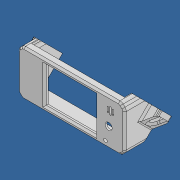
# Autodesk Inventor part: Print_Parts_TFT
Saved by Autodesk Inventor 2020 (Build 240168000, 168)
## iProperties
Created: 2020-11-15
Part Number: Print_Parts_TFT
Material: 一般
Document SubType Name: Modeling
Designer: kenta iguchi
Density: 1 g/cm^3
Appearance: 既定
Author: kenta iguchi
Autodesk Inventor part; units mm, degrees
ref_plane "YZ Plane" through (0, 0, 0) normal (1, 0, 0) x (0, 1, 0)
ref_plane "XZ Plane" through (0, 0, 0) normal (0, 1, 0) x (-1, 0, 0)
ref_plane "XY Plane" through (0, 0, 0) normal (0, 0, 1) x (1, 0, 0)
sketch "スケッチ1" plane through (0, 0, 0) normal (0, 0, 1) x (1, 0, 0)
  line L0 (28.75, -20.25) -> (-28.75, -20.25)
  line L1 (-28.75, -20.25) -> (-28.75, 20.25)
  line L2 (-28.75, 20.25) -> (28.75, 20.25)
  line L3 (28.75, 20.25) -> (28.75, -20.25)
  line L4 (28.75, -20.25) -> (-28.75, 20.25) construction
  line L5 (-28.75, -20.25) -> (28.75, 20.25) construction
  line L6 (-51.1, -23) -> (53.9, -23)
  line L7 (53.9, -23) -> (53.9, 23)
  line L8 (53.9, 23) -> (-51.1, 23)
  line L9 (-51.1, 23) -> (-51.1, -23)
  line L10 (-51.1, -23) -> (53.9, 23) construction
  line L11 (53.9, -23) -> (-51.1, 23) construction
  point P0 (0, 0)
  point P1 (1.4, 0)
  point P2 (1.4, 0)
  point P3 (0, 0)
  dimension "d0" = 40.5
  dimension "d1" = 57.5
  dimension "d2" = 51.1
  dimension "d4" = 53.9
  dimension "d5" = 46
  constraints: 24 end point, 6 midpoint, 4 parallel, 2 horizontal, 2 perpendicular, 1 horizontal alignment
  measures "d0" distance of L2.end L0.start
  measures "d1" distance of L0.start L0.end
  measures "d2" distance from line of point (0, 0) L9
  measures "d4" distance from line of L7 point (0, 0)
  measures "d5" distance of L6.end L7.end
extrude "押し出し1" add sketch "スケッチ1" against normal blind 4
sketch "スケッチ2" plane through (0, 0, 0) normal (0, 0, 1) x (1, 0, 0)
  line L0 (53.9, 23) -> (-51.1, 23) projected
  line L1 (-48.64, 20.575) -> (51.44, 20.575)
  line L2 (51.44, 20.575) -> (51.44, -20.575)
  line L3 (51.44, -20.575) -> (-48.64, -20.575)
  line L4 (-48.64, -20.575) -> (-48.64, 20.575)
  line L5 (-51.1, 23) -> (53.9, 23) projected
  point P0 (0, 0)
  point P1 (51.44, 0)
  point P2 (1.4, 23)
  point P3 (1.4, 20.575)
  point P4 (1.4, 23)
  dimension "d8" = 100.08
  dimension "d9" = 41.15
  constraints: 8 end point, 4 midpoint, 2 parallel, 1 horizontal, 1 horizontal alignment, 1 perpendicular, 1 vertical alignment
  measures "d8" distance of L2.end L3.end
  measures "d9" distance of L1.end L2.end
hole "穴1" at (51.44, 20.575, 0) at (51.44, -20.575, 0) at (-48.64, -20.575, 0) at (-48.64, 20.575, 0) direction (0, 0, -1) diameter 4.3 depth 8 tip angle 118
sketch "スケッチ3" plane through (0, 0, 0) normal (0, 0, 1) x (1, 0, 0)
  line L0 (53.9, -23) -> (53.9, 23) projected
  circle A0 centre (40.44, -19.31) radius 2
  line L1 (-51.1, -23) -> (53.9, -23) projected
  point P0 (0, 0)
  dimension "d18" = 13.46
  dimension "d19" = 4
  dimension "d26" = 3.69
  constraints: 1 centre point, 1 coincident
  measures "d18" distance from line of point (40.44, -19.31) L0
  measures "d19" diameter of A0
  measures "d26" distance from line of point (40.44, -19.31) L1
extrude "押し出し2" cut sketch "スケッチ3" against normal blind 10
sketch "スケッチ4" plane through (0, 0, -4) normal (0, 0, -1) x (-1, 0, 0)
  circle A0 centre (-40.44, -19.31) radius 2 projected
  line L0 (-37.34, -16.21) -> (-43.54, -16.21)
  line L1 (-43.54, -16.21) -> (-43.54, -22.41)
  line L2 (-43.54, -22.41) -> (-37.34, -22.41)
  line L3 (-37.34, -22.41) -> (-37.34, -16.21)
  line L4 (-37.34, -16.21) -> (-43.54, -22.41) construction
  line L5 (-43.54, -16.21) -> (-37.34, -22.41) construction
  point P0 (0, 0)
  dimension "d22" = 6.2
  dimension "d23" = 6.2
  constraints: 12 end point, 2 midpoint, 2 parallel, 1 horizontal, 1 perpendicular
  measures "d22" distance of L2.end L1.end
  measures "d23" distance of L1.end L0.end
extrude "押し出し3" cut sketch "スケッチ4" against normal blind 1
sketch "スケッチ5" plane through (0, 0, 0) normal (0, 0, 1) x (1, 0, 0)
  line L0 (-51.1, -23) -> (53.9, -23) projected
  line L1 (53.9, -23) -> (53.9, 23) projected
  circle A0 centre (44.08, -3.68) radius 4
  point P0 (0, 0)
  dimension "d27" = 19.32
  dimension "d28" = 9.82
  dimension "d29" = 8
  constraints: 1 centre point, 1 coincident
  measures "d27" distance from line of point (44.08, -3.68) L0
  measures "d28" distance from line of point (44.08, -3.68) L1
  measures "d29" diameter of A0
extrude "押し出し4" cut sketch "スケッチ5" against normal through all
chamfer "面取り1" distance 2 angle 45 4 edges at (-28.75, 0, 0) (0, 20.25, 0) (28.75, 0, 0) (0, -20.25, 0)
sketch "スケッチ6" plane through (0, 0, -4) normal (0, 0, -1) x (-1, 0, 0)
  circle A0 centre (-44.08, -3.68) radius 4 projected
  line L0 (-50.58, -10.18) -> (-37.58, -10.18)
  line L1 (-37.58, -10.18) -> (-37.58, 2.82)
  line L2 (-37.58, 2.82) -> (-50.58, 2.82)
  line L3 (-50.58, 2.82) -> (-50.58, -10.18)
  line L4 (-50.58, -10.18) -> (-37.58, 2.82) construction
  line L5 (-37.58, -10.18) -> (-50.58, 2.82) construction
  point P0 (0, 0)
  dimension "d35" = 13
  dimension "d36" = 13
  constraints: 12 end point, 2 midpoint, 2 parallel, 1 horizontal, 1 perpendicular
  measures "d35" distance of L2.end L1.end
  measures "d36" distance of L1.end L0.end
extrude "押し出し5" cut sketch "スケッチ6" against normal blind 2
sketch "スケッチ7" plane through (0, 0, 0) normal (0, 0, 1) x (1, 0, 0)
  line L0 (53.9, 23) -> (-51.1, 23)
  line L1 (53.9, -23) -> (53.9, 23)
  circle A0 centre (46.09, 12.41) radius 4.5
  line L2 (46.09, 16.91) -> (46.09, 7.91) construction
  line L3 (45.34, 16.16) -> (45.34, 8.66)
  line L4 (46.84, 8.66) -> (46.84, 16.16)
  arc A1 (46.84, 16.16) -> (45.34, 16.16) centre (46.09, 16.16) ccw
  arc A2 (45.34, 8.66) -> (46.84, 8.66) centre (46.09, 8.66) ccw
  line L5 (43.09, 15.764102) -> (43.09, 9.055898) construction
  line L6 (42.34, 15.014102) -> (42.34, 9.805898)
  line L7 (43.84, 9.805898) -> (43.84, 15.014102)
  arc A3 (43.84, 15.014102) -> (42.34, 15.014102) centre (43.09, 15.014102) ccw
  arc A4 (42.34, 9.805898) -> (43.84, 9.805898) centre (43.09, 9.805898) ccw
  line L8 (49.09, 15.764102) -> (49.09, 9.055898) construction
  line L9 (48.34, 15.014102) -> (48.34, 9.805898)
  line L10 (49.84, 9.805898) -> (49.84, 15.014102)
  arc A5 (49.84, 15.014102) -> (48.34, 15.014102) centre (49.09, 15.014102) ccw
  arc A6 (48.34, 9.805898) -> (49.84, 9.805898) centre (49.09, 9.805898) ccw
  point P0 (0, 0)
  point P1 (43.09, 12.41)
  point P2 (49.09, 12.41)
  dimension "d39" = 7.81
  dimension "d40" = 10.59
  dimension "d41" = 9
  dimension "d42" = 1.5
  dimension "d43" = 1.5
  dimension "d44" = 1.5
  dimension "d45" = 3
  dimension "d46" = 6
  constraints: 24 end point, 24 point on circle, 12 tangent, 7 centre point, 6 point on line, 4 parallel, 3 midpoint, 2 coincident, 2 vertical
  measures "d39" distance from line of point (46.09, 12.41) L1
  measures "d40" distance from line of point (46.09, 12.41) L0
  measures "d41" diameter of A0
  measures "d42" diameter of A2
  measures "d43" diameter of A4
  measures "d44" diameter of A6
  measures "d45" distance of A0.centre point (43.09, 12.41)
  measures "d46" distance between parallel lines of L8 L5
extrude "押し出し6" cut sketch "スケッチ7" against normal blind 10 contours L10 A0 A6 L9 A5 | A0 A5 L10 | L10 A6 A0 | A1 L4 A2 L3 | A3 L7 A4 A0 L6 | A0 L6 A3 | A4 L6 A0
sketch "スケッチ8" plane through (0, 0, -4) normal (0, 0, -1) x (-1, 0, 0)
  line L0 (-48.34, 15.014102) -> (-48.34, 9.805898)
  arc A0 (-49.84, 9.805898) -> (-48.34, 9.805898) centre (-49.09, 9.805898) ccw
  line L1 (-49.84, 9.805898) -> (-49.84, 15.014102)
  arc A1 (-48.34, 15.014102) -> (-49.84, 15.014102) centre (-49.09, 15.014102) ccw
  line L2 (-46.84, 8.66) -> (-46.84, 16.16)
  arc A2 (-45.34, 16.16) -> (-46.84, 16.16) centre (-46.09, 16.16) ccw
  line L3 (-45.34, 16.16) -> (-45.34, 8.66)
  arc A3 (-46.84, 8.66) -> (-45.34, 8.66) centre (-46.09, 8.66) ccw
  line L4 (-42.34, 15.014102) -> (-42.34, 9.805898)
  arc A4 (-43.84, 9.805898) -> (-42.34, 9.805898) centre (-43.09, 9.805898) ccw
  line L5 (-43.84, 9.805898) -> (-43.84, 15.014102)
  arc A5 (-42.34, 15.014102) -> (-43.84, 15.014102) centre (-43.09, 15.014102) ccw
  line L6 (-46.09, 8.66) -> (-46.09, 16.16)
  circle A6 centre (-46.09, 12.41) radius 5
  point P0 (0, 0)
  dimension "d49" = 10
  constraints: 2 end point, 1 centre point, 1 coincident, 1 midpoint, 1 vertical
  measures "d49" diameter of A6
extrude "押し出し7" cut sketch "スケッチ8" against normal blind 2
sketch "スケッチ9" plane through (0, 0, 0) normal (0, 0, 1) x (1, 0, 0)
  line L0 (53.9, 23) -> (-51.1, 23) projected
  line L1 (-51.1, 23) -> (-51.1, -23) projected
  line L2 (-51.1, -23) -> (53.9, -23) projected
  line L3 (53.9, -23) -> (53.9, 23) projected
  line L4 (-54.1, 26) -> (56.9, 26)
  line L5 (56.9, 26) -> (56.9, -26)
  line L6 (56.9, -26) -> (-54.1, -26)
  line L7 (-54.1, -26) -> (-54.1, 26)
  circle A0 centre (51.44, 20.575) radius 2.15 projected
  circle A1 centre (51.44, 20.575) radius 4
  point P0 (0, 0)
  dimension "d52" = 3
  dimension "d67" = 8
  constraints: 8 end point, 1 centre point, 1 coincident, 3 other
  measures "d52" distance between parallel lines of L0 L4
  measures "d67" diameter of A1
extrude "押し出し8" add sketch "スケッチ9" against normal up to surface (4 mm away) contours L0 A1 L3 | L4 L5 L6 L7 picked at (50.3712, 23.236403)
sketch "スケッチ10" plane through (0, 0, -4) normal (0, 0, -1) x (-1, 0, 0)
  circle A0 centre (48.64, -20.575) radius 2.15 projected
  circle A1 centre (-51.44, 20.575) radius 2.15 projected
  circle A2 centre (48.64, 20.575) radius 2.15 projected
  circle A3 centre (-51.44, 20.575) radius 2.2
  circle A4 centre (48.64, 20.575) radius 2.2
  circle A5 centre (48.64, -20.575) radius 2.2
  circle A6 centre (-51.44, -20.575) radius 2.15 projected
  circle A7 centre (-51.44, -20.575) radius 2.2
  circle A8 centre (-51.44, 20.575) radius 2.15 projected
  circle A9 centre (-51.44, 20.575) radius 4
  circle A10 centre (48.64, 20.575) radius 4
  circle A11 centre (48.64, -20.575) radius 4
  circle A12 centre (-51.44, -20.575) radius 4
  point P0 (0, 0)
  dimension "d55" = 4.4
  dimension "d56" = 4.4
  dimension "d57" = 4.4
  dimension "d58" = 4.4
  dimension "d59" = 8
  dimension "d60" = 8
  dimension "d61" = 8
  dimension "d62" = 8
  constraints: 8 centre point, 8 coincident
  measures "d55" diameter of A3
  measures "d56" diameter of A4
  measures "d57" diameter of A5
  measures "d58" diameter of A7
  measures "d59" diameter of A9
  measures "d60" diameter of A10
  measures "d61" diameter of A11
  measures "d62" diameter of A12
extrude "押し出し9" add sketch "スケッチ10" along normal blind 3 contours A9 | A10 | A11 | A12
sketch "スケッチ11" plane through (0, 0, 0) normal (0, 0, 1) x (1, 0, 0)
  circle A0 centre (-48.64, 20.575) radius 2.15 projected
  circle A1 centre (51.44, -20.575) radius 2.15 projected
  circle A2 centre (51.44, 20.575) radius 2.15 projected
  circle A3 centre (-48.64, -20.575) radius 2.15 projected
  point P0 (0, 0)
extrude "押し出し10" add sketch "スケッチ11" against normal up to surface (4 mm away)
sketch "スケッチ12" plane through (0, 0, -4) normal (0, 0, -1) x (-1, 0, 0)
  circle A0 centre (48.64, 20.575) radius 4 projected
  circle A1 centre (-51.44, 20.575) radius 4 projected
  circle A2 centre (48.64, -20.575) radius 4 projected
  circle A3 centre (-51.44, -20.575) radius 4 projected
  line L0 (54.1, 26) -> (54.1, -26) projected
  line L1 (-56.9, 26) -> (54.1, 26) projected
  line L2 (-56.9, -26) -> (-56.9, 26) projected
  line L3 (54.1, -26) -> (-56.9, -26) projected
  line L4 (51.3, 23.2) -> (51.3, -23.2)
  line L5 (51.3, -23.2) -> (-54.1, -23.2)
  line L6 (-54.1, -23.2) -> (-54.1, 23.2)
  line L7 (-54.1, 23.2) -> (51.3, 23.2)
  circle A4 centre (-51.44, 20.575) radius 4 projected
  circle A5 centre (-51.44, 20.575) radius 2.2 projected
  circle A6 centre (48.64, 20.575) radius 2.2 projected
  circle A7 centre (48.64, -20.575) radius 2.2 projected
  circle A8 centre (-51.44, -20.575) radius 2.2 projected
  point P0 (0, 0)
  point P1 (-48.421826, 23.2)
  point P2 (45.621826, 23.2)
  point P3 (51.3, 17.587627)
  point P4 (51.3, -17.587627)
  point P5 (45.621826, -23.2)
  point P6 (-48.421826, -23.2)
  point P7 (-54.1, -17.587627)
  point P8 (-54.1, 17.587627)
  dimension "d68" = 2.8
  constraints: 8 end point, 3 other
  measures "d68" distance between parallel lines of L1 L7
extrude "押し出し11" add sketch "スケッチ12" along normal blind 4 contours L0 L3 L2 L1
sketch "スケッチ13" plane through (51.44, 20.575, -4) normal (0, 0, -1) x (-1, 0, 0)
  circle A0 centre (0, 0) radius 2.2 projected
  circle A1 centre (0, -41.15) radius 2.2 projected
  circle A2 centre (100.08, -41.15) radius 2.2 projected
  circle A3 centre (100.08, 0) radius 2.2 projected
  point P0 (51.44, -20.575)
extrude "押し出し12" cut sketch "スケッチ13" against normal blind 2
sketch "スケッチ14" plane through (0, 0, -8) normal (0, 0, -1) x (-1, 0, 0)
  line L0 (54.1, -26) -> (54.1, 26)
  line L1 (-56.9, 26) -> (-56.9, -26)
  line L2 (-54.1, -17.587627) -> (-54.1, 17.587627)
  line L3 (51.3, 17.587627) -> (51.3, -17.587627)
  line L4 (-56.9, 26) -> (54.1, 26)
  line L5 (54.1, 26) -> (59.3, 26)
  line L6 (59.3, 26) -> (59.3, -26)
  line L7 (59.3, -26) -> (54.1, -26)
  line L8 (54.1, -26) -> (54.1, 26)
  line L9 (-56.9, 26) -> (-62.1, 26)
  line L10 (-62.1, 26) -> (-62.1, -26)
  line L11 (-62.1, -26) -> (-56.9, -26)
  line L12 (-56.9, -26) -> (-56.9, 26)
  point P0 (0, 0)
  point P1 (-56.9, -26)
  dimension "d80" = 8
  dimension "d81" = 8
  constraints: 16 end point, 4 parallel, 2 horizontal, 2 perpendicular, 1 coincident, 1 horizontal alignment, 1 point on line
  measures "d80" distance between parallel lines of L6 L3
  measures "d81" distance between parallel lines of L10 L2
extrude "押し出し13" add sketch "スケッチ14" against normal up to surface (8 mm away)
sketch "スケッチ16" plane through (0, 0, -8) normal (0, 0, -1) x (-1, 0, 0)
  line L0 (59.3, 26) -> (-62.1, 26)
  line L1 (-62.1, 26) -> (-62.1, -26)
  line L2 (-62.1, -26) -> (59.3, -26)
  line L3 (59.3, -26) -> (59.3, 26)
  arc A0 (45.621826, -23.2) -> (51.3, -17.587627) centre (48.64, -20.575) ccw
  arc A1 (-54.1, -17.587627) -> (-48.421826, -23.2) centre (-51.44, -20.575) ccw
  line L4 (-54.1, -17.587627) -> (-54.1, 17.587627)
  arc A2 (-48.421826, 23.2) -> (-54.1, 17.587627) centre (-51.44, 20.575) ccw
  arc A3 (51.3, 17.587627) -> (45.621826, 23.2) centre (48.64, 20.575) ccw
  line L5 (51.3, 17.587627) -> (51.3, -17.587627)
  line L6 (-62.1, 26) -> (-54.1, 26)
  line L7 (-54.1, 26) -> (-54.1, -26)
  line L8 (-54.1, -26) -> (-62.1, -26)
  line L9 (-62.1, -26) -> (-62.1, 26)
  line L10 (-62.1, 26) -> (59.3, 26)
  line L11 (59.3, 26) -> (51.3, 26)
  line L12 (51.3, 26) -> (51.3, -26)
  line L13 (51.3, -26) -> (59.3, -26)
  line L14 (59.3, -26) -> (59.3, 26)
  point P0 (0, 0)
  point P1 (51.3, -23.562373)
  point P2 (51.3, 23.562373)
  point P3 (-54.1, 23.562373)
  point P4 (-54.1, -23.562373)
  constraints: 16 end point, 4 parallel, 2 horizontal, 2 perpendicular, 2 point on line, 2 vertical alignment
extrude "押し出し14" add sketch "スケッチ16" along normal blind 10 contours L3 L2 L12 A0 L5 A3 L0 | L7 A2 L4 A1 L2 L1 L0
chamfer "面取り4" distance 2 angle 45 2 edges at (58.1, 26, -18) (-55.3, 26, -18)
sketch "スケッチ17" plane through (-59.3, -26, 0) normal (-1, 0, 0) x (0, 0, 1)
  line L0 (-18, 50) -> (-16, 52) projected
  line L1 (-18, 0) -> (-18, 50) projected
  line L2 (0, 0) -> (-18, 0) projected
  line L3 (-18, 50) -> (-68, 0)
  line L4 (-8, 0) -> (-18, 0) projected
  line L5 (-68, 0) -> (-18, 0)
  line L6 (-18, 0) -> (0, 0) projected
  line L7 (-18, 0) -> (-43, 25)
  point P0 (0, 26)
  constraints: 6 end point, 2 collinear, 1 midpoint
extrude "押し出し15" add sketch "スケッチ17" against normal up to surface (8 mm away) contours L7 L3 L1
sketch "スケッチ18" plane through (62.1, -26, 0) normal (1, 0, 0) x (0, 0, -1)
  line L0 (18, 50) -> (18, 0)
  line L1 (4, 8.412373) -> (4, 43.587627)
  line L2 (7, 8.412373) -> (4, 8.412373)
  line L3 (7, 8.412373) -> (18, 8.412373)
  line L4 (18, 2.437627) -> (18, 8.412373)
  line L5 (8, 2.437627) -> (18, 2.437627)
  line L6 (8, 0) -> (18, 0)
  line L7 (43, 25) -> (18, 0)
  line L8 (16, 52) -> (43, 25)
  line L9 (18, 43.587627) -> (18, 49.562373)
  line L10 (7, 43.587627) -> (18, 43.587627)
  line L11 (4, 43.587627) -> (7, 43.587627)
  line L12 (8, 0) -> (8, 2.437627)
  line L13 (8, 52) -> (16, 52)
  line L14 (8, 49.562373) -> (8, 52)
  line L15 (8, 49.562373) -> (18, 49.562373)
  point P0 (0, 26)
  point P1 (18, 50)
  point P2 (18, 8.412373)
  point P3 (18, 0)
extrude "押し出し16" add sketch "スケッチ18" against normal up to surface (8 mm away) contours L8 L7 L0
sketch "スケッチ20" plane through (-59.3, -26, 0) normal (-1, 0, 0) x (0, 0, 1)
  line L0 (0, 0) -> (-18, 0) projected
  line L1 (0, 0) -> (0, 52) projected
  line L2 (-8.6, 38.36) -> (-11.5, 38.36)
  line L3 (-11.5, 38.36) -> (-11.5, 11.86)
  line L4 (-11.5, 11.86) -> (-8.6, 11.86)
  line L5 (-8.6, 11.86) -> (-8.6, 38.36)
  point P0 (0, 26)
  dimension "d96" = 8.6
  dimension "d97" = 2.9
  dimension "d98" = 11.86
  dimension "d99" = 38.36
  constraints: 8 end point, 2 parallel, 1 horizontal, 1 perpendicular
  measures "d96" distance between parallel lines of L1 L5
  measures "d97" distance of L3.end L4.end
  measures "d98" distance between parallel lines of L0 L4
  measures "d99" distance between parallel lines of L0 L2
extrude "押し出し18" cut sketch "スケッチ20" against normal blind 10
sketch "スケッチ21" plane through (-59.3, -26, 0) normal (-1, 0, 0) x (0, 0, 1)
  line L0 (-8.6, 38.36) -> (-8.6, 11.86) projected
  line L1 (-8.6, 11.86) -> (-11.5, 11.86) projected
  line L2 (-11.5, 11.86) -> (-11.5, 38.36) projected
  line L3 (-11.5, 38.36) -> (-8.6, 38.36) projected
  line L4 (-12.5, 10.86) -> (-7.6, 10.86)
  line L5 (-7.6, 10.86) -> (-7.6, 39.36)
  line L6 (-7.6, 39.36) -> (-12.5, 39.36)
  line L7 (-12.5, 39.36) -> (-12.5, 10.86)
  point P0 (0, 26)
  dimension "d102" = 1
  constraints: 8 end point, 3 other
  measures "d102" distance between parallel lines of L1 L4
extrude "押し出し19" cut sketch "スケッチ21" against normal blind 10
fillet "フィレット2" radius 1 4 edges at (-55.3, 13.36, -12.5) (-55.3, 13.36, -7.6) (-55.3, -15.14, -12.5) (-55.3, -15.14, -7.6)
sketch "スケッチ24" plane through (62.1, 26, -16) normal (0, 0.7071068, -0.7071068) x (-1, 0, 0)
  line L0 (0, 0) -> (0, -38.183766)
  line L1 (0, -38.183766) -> (-12, -38.183766)
  line L2 (-12, -38.183766) -> (-12, -18.183766)
  line L3 (-12, -18.183766) -> (0, -18.183766)
  line L4 (0, -18.183766) -> (0, -38.183766)
  line L5 (113.4, 0) -> (113.4, -38.183766)
  line L6 (121.4, -38.183766) -> (121.4, 0)
  line L7 (121.4, 0) -> (113.4, 0)
  line L8 (121.4, -38.183766) -> (121.4, 0)
  line L9 (121.4, -38.183766) -> (133.4, -38.183766)
  line L10 (133.4, -38.183766) -> (133.4, -18.183766)
  line L11 (133.4, -18.183766) -> (121.4, -18.183766)
  line L12 (121.4, -18.183766) -> (121.4, -38.183766)
  line L13 (121.4, -38.183766) -> (113.4, -38.183766)
  point P0 (62.1, -7.071068)
  point P1 (0, -18.183766)
  point P2 (8, -38.183766)
  dimension "d118" = 12
  dimension "d119" = 20
  dimension "d120" = 12
  dimension "d121" = 20
  constraints: 16 end point, 4 parallel, 2 horizontal, 2 horizontal alignment, 2 perpendicular
  measures "d118" distance of L2.end L3.end
  measures "d119" distance of L1.end L2.end
  measures "d120" distance of L11.end L10.end
  measures "d121" distance of L10.end L9.end
extrude "押し出し21" add sketch "スケッチ24" against normal blind 5 contours L0 L1 L2 L3 | L6 L11 L10 L9
chamfer "面取り6" distance 12 angle 45 2 edges at (62.1, 2.5355, -32.3934) (-59.3, 2.5355, -32.3934)
chamfer "面取り7" distance 5 angle 45 4 edges at (62.1, -26, -9) (-59.3, -26, -9) (62.1, 26, -8) (-59.3, 26, -8)
fillet "フィレット3" radius 5 8 edges at (-59.3, 21, -10.5) (-54.3, 26, -8) (-59.3, -21, -11.5) (-54.3, -26, -9) (57.1, -26, -9) (62.1, -21, -11.5) (62.1, 21, -10.5) (57.1, 26, -8)
chamfer "面取り8" distance 2 angle 45 8 edges at (74.1, 9.6066, -25.3223) (74.1, 11.3744, -27.0901) (74.1, -4.5355, -39.4645) (74.1, -2.7678, -41.2322) (-71.3, 9.6066, -25.3223) (-71.3, 11.3744, -27.0901) (-71.3, -4.5355, -39.4645) (-71.3, -2.7678, -41.2322)
fillet "フィレット4" radius 2 12 edges at (-59.3, -5.9497, -23.9082) (62.1, -5.9497, -23.9082) (72.1, 10.6673, -26.383) (74.1, 9.9602, -28.5043) (74.1, -1.3536, -39.818) (72.1, -3.4748, -40.5252) (-69.3, -3.4748, -40.5252) (-71.3, -1.3536, -39.818) (-71.3, 9.9602, -28.5043) (-69.3, 10.6673, -26.383) (62.1, 7.1318, -22.8475) (-59.3, 7.1318, -22.8475)
chamfer "面取り9" distance 2 angle 45 16 edges at (-58.9194, 20.8423, 0) (-56.8, 23.5, 0) (-54.1423, 25.6194, 0) (1.4, 26, 0) (56.9423, 25.6194, 0) (59.6, 23.5, 0) (61.7194, 20.8423, 0) (62.1, 0, 0) (61.7194, -20.8423, 0) (59.6, -23.5, 0) (56.9423, -25.6194, 0) (1.4, -26, 0) (-54.1423, -25.6194, 0) (-56.8, -23.5, 0) (-58.9194, -20.8423, 0) (-59.3, 0, 0)
sketch "スケッチ26" plane through (51.44, 20.575, -18) normal (0, 0, 1) x (1, 0, 0)
  arc A0 (2.66, -2.987373) -> (2.66, 2.987373) centre (0, 0) ccw
  line L0 (2.66, 2.987373) -> (2.66, -2.987373)
  arc A1 (2.66, -44.137373) -> (2.66, -38.162627) centre (0, -41.15) ccw
  line L1 (2.66, -38.162627) -> (2.66, -44.137373)
  arc A2 (-102.74, 2.987373) -> (-102.74, -2.987373) centre (-100.08, 0) ccw
  line L2 (-102.74, -2.987373) -> (-102.74, 2.987373)
  arc A3 (-102.74, -38.162627) -> (-102.74, -44.137373) centre (-100.08, -41.15) ccw
  line L3 (-102.74, -44.137373) -> (-102.74, -38.162627)
  point P0 (-51.44, -20.575)
extrude "押し出し22" cut sketch "スケッチ26" against normal blind 10
sketch "スケッチ27" plane through (0, 0, -8) normal (0, 0, -1) x (-1, 0, 0)
  line L0 (51.3, -26) -> (51.3, -23.562373)
  arc A0 (45.621826, -23.2) -> (51.3, -23.562373) centre (48.64, -20.575) ccw
  line L1 (45.621826, -23.2) -> (-48.421826, -23.2)
  arc A1 (-54.1, -23.562373) -> (-48.421826, -23.2) centre (-51.44, -20.575) ccw
  line L2 (-54.1, -23.562373) -> (-54.1, -26)
  line L3 (-54.1, -26) -> (51.3, -26)
  point P0 (0, 0)
extrude "押し出し23" add sketch "スケッチ27" along normal up to surface surface through (62.1, -1, -43) normal (0, -0.7071068, -0.7071068)
ref_plane "作業平面2" through (-61.3, -1, -14.715729) normal (0, 0.7071068, -0.7071068) x (-1, 0, 0)
sketch "スケッチ29" plane through (-61.3, -1, -14.715729) normal (0, 0.7071068, -0.7071068) x (-1, 0, 0)
  arc A0 (8.585786, -0.585786) -> (7.171573, 0) centre (7.171573, -2) ccw
  line L0 (9.414214, -1.414214) -> (8.585786, -0.585786)
  arc A1 (10, -2.828427) -> (9.414214, -1.414214) centre (8, -2.828427) ccw
  line L1 (10, -2.828427) -> (10, -17.171573)
  arc A2 (9.414214, -18.585786) -> (10, -17.171573) centre (8, -17.171573) ccw
  line L2 (8.585786, -19.414214) -> (9.414214, -18.585786)
  arc A3 (7.171573, -20) -> (8.585786, -19.414214) centre (7.171573, -18) ccw
  line L3 (7.171573, -20) -> (-1.414214, -20)
  line L4 (-1.414214, -20) -> (-1.414214, 0.585786)
  arc A4 (-1.414214, 0.585786) -> (0, 0) centre (0, 2) ccw
  line L5 (0, 0) -> (7.171573, 0)
  arc A5 (-133.985786, -19.414214) -> (-132.571573, -20) centre (-132.571573, -18) ccw
  line L6 (-134.814214, -18.585786) -> (-133.985786, -19.414214)
  arc A6 (-135.4, -17.171573) -> (-134.814214, -18.585786) centre (-133.4, -17.171573) ccw
  line L7 (-135.4, -17.171573) -> (-135.4, -2.828427)
  arc A7 (-134.814214, -1.414214) -> (-135.4, -2.828427) centre (-133.4, -2.828427) ccw
  line L8 (-133.985786, -0.585786) -> (-134.814214, -1.414214)
  arc A8 (-132.571573, 0) -> (-133.985786, -0.585786) centre (-132.571573, -2) ccw
  line L9 (-132.571573, 0) -> (-125.4, 0)
  arc A9 (-125.4, 0) -> (-123.985786, 0.585786) centre (-125.4, 2) ccw
  line L10 (-123.985786, -20) -> (-123.985786, 0.585786)
  line L11 (-123.985786, -20) -> (-132.571573, -20)
  point P0 (-61.3, 11.112698)
  point P1 (-129.4, -10)
  point P2 (4, -10)
  dimension "d152" = 10
  dimension "d153" = 6
  dimension "d154" = 6
  constraints: 1 horizontal alignment
  measures "d152" distance from line of L11 point (-129.4, -10)
  measures "d153" distance from line of point (4, -10) L1
  measures "d154" distance from line of point (-129.4, -10) L7
hole "穴3" at (68.1, -8.071068, -21.786797) at (-65.3, -8.071068, -21.786797) direction (0, 0.7071068, -0.7071068) diameter 4.3 depth 33.75 counterbore diameter 8 counterbore depth 15
sketch "スケッチ30" plane through (-61.3, -1, -14.715729) normal (0, 0.7071068, -0.7071068) x (-1, 0, 0)
  circle A0 centre (4, -10) radius 4
  arc A1 (8.585786, -0.585786) -> (7.171573, 0) centre (7.171573, -2) ccw
  line L0 (9.414214, -1.414214) -> (8.585786, -0.585786)
  arc A2 (10, -2.828427) -> (9.414214, -1.414214) centre (8, -2.828427) ccw
  line L1 (10, -2.828427) -> (10, -17.171573)
  arc A3 (9.414214, -18.585786) -> (10, -17.171573) centre (8, -17.171573) ccw
  line L2 (8.585786, -19.414214) -> (9.414214, -18.585786)
  arc A4 (7.171573, -20) -> (8.585786, -19.414214) centre (7.171573, -18) ccw
  line L3 (7.171573, -20) -> (-1.414214, -20)
  line L4 (-1.414214, -20) -> (-1.414214, 0.585786)
  arc A5 (-1.414214, 0.585786) -> (0, 0) centre (0, 2) ccw
  line L5 (0, 0) -> (7.171573, 0)
  circle A6 centre (-129.4, -10) radius 4
  arc A7 (-133.985786, -19.414214) -> (-132.571573, -20) centre (-132.571573, -18) ccw
  line L6 (-134.814214, -18.585786) -> (-133.985786, -19.414214)
  arc A8 (-135.4, -17.171573) -> (-134.814214, -18.585786) centre (-133.4, -17.171573) ccw
  line L7 (-135.4, -17.171573) -> (-135.4, -2.828427)
  arc A9 (-134.814214, -1.414214) -> (-135.4, -2.828427) centre (-133.4, -2.828427) ccw
  line L8 (-133.985786, -0.585786) -> (-134.814214, -1.414214)
  arc A10 (-132.571573, 0) -> (-133.985786, -0.585786) centre (-132.571573, -2) ccw
  line L9 (-132.571573, 0) -> (-125.4, 0)
  arc A11 (-125.4, 0) -> (-123.985786, 0.585786) centre (-125.4, 2) ccw
  line L10 (-123.985786, -20) -> (-123.985786, 0.585786)
  line L11 (-123.985786, -20) -> (-132.571573, -20)
  line L12 (17.830509, -6) -> (-146.954567, -6)
  line L13 (-146.954567, -6) -> (-146.954567, -14)
  line L14 (-146.954567, -14) -> (17.830509, -14)
  line L15 (17.830509, -14) -> (17.830509, -6)
  point P0 (-61.3, 11.112698)
  point P1 (-135.4, -14)
  point P2 (-129.4, -14)
  point P3 (-129.4, -6)
  point P4 (-135.4, -6)
  point P5 (4, -14)
  point P6 (10, -14)
  point P7 (10, -6)
  point P8 (4, -6)
  constraints: 8 end point, 2 parallel, 2 tangent, 1 horizontal, 1 perpendicular
extrude "押し出し24" cut sketch "スケッチ30" along normal up to surface (15 mm away) contours A0 L12 L1 L14 | A6 L14 L7 L12
chamfer "面取り10" distance 2 angle 45 6 edges at (-61.3, -4.5355, -25.3224) (-68.3, -2.4141, -33.1006) (-68.3, 3.2427, -27.4437) (71.1, 3.2427, -27.4437) (64.1, -4.5355, -25.3224) (71.1, -2.4141, -33.1006)
